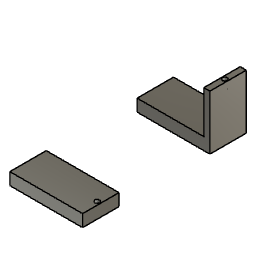
夹钳 (Autodesk Fusion 360 design; units mm, degrees)
Autodesk Fusion 360 part; units mm, degrees
sketch "草图1" plane through (0, 0, 0) normal (0, 0, 1) x (1, 0, 0)
  line L0 (0, 15) -> (6, 15)
  line L1 (6, 15) -> (6, 12)
  line L2 (6, 12) -> (0, 12)
  line L3 (0, 12) -> (0, 15)
  constraint horizontal L0
  constraint vertical L1
  constraint horizontal L2
  constraint vertical L3
extrude "拉伸1" add sketch "草图1" along normal blind 1 makes body 1
sketch "草图2" plane through (0, 0, 0) normal (0, 0, 1) x (1, 0, 0)
  line L0 (0, 1.5) -> (6, 1.5)
  line L1 (6, 1.5) -> (6, 4.5)
  line L2 (6, 4.5) -> (0, 4.5)
  line L3 (0, 4.5) -> (0, 1.5)
  constraint horizontal L0
  constraint vertical L1
  constraint horizontal L2
  constraint vertical L3
extrude "拉伸2" add sketch "草图2" along normal blind 1 separate body makes body 2
sketch "草图3" plane through (0, 0, 1) normal (0, 0, 1) x (-1, 0, 0)
  line L0 (0, -12) -> (-6, -12)
  line L1 (-6, -12) -> (-6, -15)
  line L2 (-6, -15) -> (0, -15)
  line L3 (0, -15) -> (0, -12)
  line L4 (-5.5029, -15) -> (-6, -15)
  line L5 (-6, -15) -> (-6, -12)
  line L6 (-6, -12) -> (-5.5029, -12)
  line L7 (-5.5029, -12) -> (-5.5029, -15)
  constraint horizontal L4
  constraint vertical L5
  constraint horizontal L6
  constraint vertical L7
  constraint coincident L0.end L1.start
  constraint coincident L2 L4.start
extrude "拉伸3" add sketch "草图3" along normal blind 3.5 contours L0 L1 L2 L4 L5 L6 L7 bodies 1
hole "孔1" at (5.7503, 13.4785, 4.5) direction (0, 0, -1) diameter 0.4 depth 0.6 tip angle 118 bodies 1
hole "孔2" at (5.7198, 2.9769, 1) direction (0, 0, -1) diameter 0.4 depth 1 tip angle 118 bodies 2
